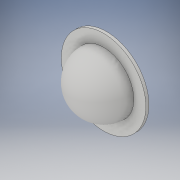
# Autodesk Inventor part: DomeTest
Saved by Autodesk Inventor 2018 (Build 220112000, 112)
## iProperties
Created: 2019-02-18
Part Number: DomeTest
Material: Generic
Document SubType Name: Modeling
Designer: anirudh
Density: 1 g/cm^3
Appearance: Default
Author: anirudh
Autodesk Inventor part; units mm, degrees
ref_plane "YZ Plane" through (0, 0, 0) normal (1, 0, 0) x (0, 1, 0)
ref_plane "XZ Plane" through (0, 0, 0) normal (0, 1, 0) x (-1, 0, 0)
ref_plane "XY Plane" through (0, 0, 0) normal (0, 0, 1) x (1, 0, 0)
sketch "Sketch1" plane through (0, 0, 0) normal (0, 0, 1) x (1, 0, 0)
  circle A0 centre (0, 25.4) radius 31.75
  line L0 (0, 57.15) -> (0, -6.35)
  line L1 (0, -6.35) -> (0, -21.5951)
  point P0 (0, 0)
  dimension "d5" = 63.5
  constraints: 4 end point, 2 point on circle, 1 centre point, 1 point on line, 1 vertical
  measures "d5" diameter of A0
revolve "Revolution2" add sketch "Sketch1" angle 180 about axis through (0, -6.35, 0) along (0, -1, 0) picked at (11.1905, 16.0775) contours A0 L0
sketch "Sketch3" plane through (0, 25.4, 0) normal (0, 0, -1) x (-1, 0, 0)
  circle A0 centre (0, 0) radius 44.45
  point P0 (0, -25.4)
  dimension "d7" = 88.9
  constraints: 1 centre point
  measures "d7" diameter of A0
extrude "Extrusion2" add sketch "Sketch3" along normal blind 3.175
body "Solid2"
